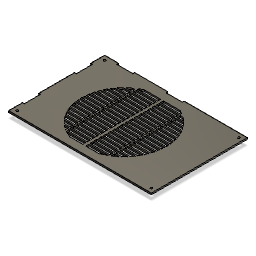
PSU and Board Enclosure (Autodesk Fusion 360 design; units mm, degrees)
Autodesk Fusion 360 part; units mm, degrees
note: some values were not read from the file. Chosen so that the rebuilt part matches the saved one: which bodies a step acts on; a direction; that a step has no effect; which face or edge a step refers to; which pieces of a blend or face edit are solid. Set by a fixed rule: which sketch regions a step uses.
(part 1 of 3)
mesh "Netz1" [no effect]
sketch "Skizze1" plane through (0, 0, 0) normal (0, 1, 0) x (1, 0, 0)
  line L0 (0, 0) -> (115, 0)
  line L1 (115, 0) -> (115, -240)
  line L2 (115, -240) -> (0, -240)
  line L3 (0, -240) -> (0, 0)
  line L4 (-7, 7) -> (122, 7)
  line L5 (122, 7) -> (122, -290)
  line L6 (122, -290) -> (-7, -290)
  line L7 (-7, -290) -> (-7, 7)
  line L8 (-9.4, 9.4) -> (124.4, 9.4)
  line L9 (124.4, 9.4) -> (124.4, -294)
  line L10 (124.4, -294) -> (-9.4, -294)
  line L11 (-9.4, -294) -> (-9.4, 9.4)
  line L12 (0, -240) -> (115, -240)
  line L13 (115, -240) -> (115, -290)
  line L14 (115, -290) -> (0, -290)
  line L15 (0, -290) -> (0, -240)
  line L16 (10, -225) -> (15, -225)
  line L17 (15, -225) -> (15, -230)
  line L18 (15, -230) -> (10, -230)
  line L19 (10, -230) -> (10, -225)
  line L20 (100, -225) -> (105, -225)
  line L21 (105, -225) -> (105, -230)
  line L22 (105, -230) -> (100, -230)
  line L23 (100, -230) -> (100, -225)
  line L24 (10, -120) -> (15, -120)
  line L25 (15, -120) -> (15, -125)
  line L26 (15, -125) -> (10, -125)
  line L27 (10, -125) -> (10, -120)
  line L28 (100, -120) -> (105, -120)
  line L29 (105, -120) -> (105, -125)
  line L30 (105, -125) -> (100, -125)
  line L31 (100, -125) -> (100, -120)
  line L32 (0, -25) -> (115, -25)
  line L33 (10, -40) -> (10, -35)
  line L34 (15, -40) -> (10, -40)
  line L35 (100, -40) -> (100, -35)
  line L36 (10, -35) -> (15, -35)
  line L37 (15, -35) -> (15, -40)
  line L38 (100, -35) -> (105, -35)
  line L39 (105, -40) -> (100, -40)
  line L40 (105, -35) -> (105, -40)
  circle A0 centre (40, -70) radius 30
  circle A1 centre (40, -70) radius 32.4
  line L41 (3.2857, -51.5) -> (78.5153, -51.5)
  line L42 (78.5153, -51.5) -> (78.5153, -56.5)
  line L43 (78.5153, -56.5) -> (3.2857, -56.5)
  line L44 (3.2857, -56.5) -> (3.2857, -51.5)
  line L45 (78.5153, -59.5) -> (78.5153, -64.5)
  line L46 (3.2857, -64.5) -> (3.2857, -59.5)
  line L47 (3.2857, -59.5) -> (78.5153, -59.5)
  line L48 (78.5153, -64.5) -> (3.2857, -64.5)
  line L49 (78.5153, -67.5) -> (78.5153, -72.5)
  line L50 (3.2857, -72.5) -> (3.2857, -67.5)
  line L51 (3.2857, -67.5) -> (78.5153, -67.5)
  line L52 (78.5153, -72.5) -> (3.2857, -72.5)
  line L53 (78.5153, -75.5) -> (78.5153, -80.5)
  line L54 (3.2857, -80.5) -> (3.2857, -75.5)
  line L55 (3.2857, -75.5) -> (78.5153, -75.5)
  line L56 (78.5153, -80.5) -> (3.2857, -80.5)
  line L57 (78.5153, -83.5) -> (78.5153, -88.5)
  line L58 (3.2857, -88.5) -> (3.2857, -83.5)
  line L59 (3.2857, -83.5) -> (78.5153, -83.5)
  line L60 (78.5153, -88.5) -> (3.2857, -88.5)
  line L61 (78.5153, -91.5) -> (78.5153, -96.5)
  line L62 (3.2857, -96.5) -> (3.2857, -91.5)
  line L63 (3.2857, -91.5) -> (78.5153, -91.5)
  line L64 (78.5153, -96.5) -> (3.2857, -96.5)
  line L65 (78.5153, -43.5) -> (78.5153, -48.5)
  line L66 (3.2857, -48.5) -> (3.2857, -43.5)
  line L67 (3.2857, -43.5) -> (78.5153, -43.5)
  line L68 (78.5153, -48.5) -> (3.2857, -48.5)
  dimension "d1" = 240
  dimension "d2" = 115
  dimension "d7" = 7
  dimension "d8" = 7
  dimension "d9" = 7
  dimension "d12" = 2.4
  dimension "d13" = 4
  dimension "d14" = 2.4
  dimension "d15" = 2.4
  dimension "d24" = 50
  dimension "d48" = 5
  dimension "d49" = 5
  dimension "d50" = 5
  dimension "d51" = 5
  dimension "d52" = 5
  dimension "d53" = 5
  dimension "d54" = 5
  dimension "d55" = 5
  dimension "d56" = 10
  dimension "d57" = 10
  dimension "d58" = 10
  dimension "d59" = 100
  dimension "d61" = 215
  dimension "d62" = 5
  dimension "d63" = 5
  dimension "d64" = 5
  dimension "d65" = 5
  dimension "d66" = 10
  dimension "d87" = 60
  dimension "d89" = 40
  dimension "d90" = 2.4
  dimension "d505" = 45
  dimension "d509" = 5
  dimension "d510" = 5
  dimension "d511" = 5
  dimension "d512" = 5
  dimension "d513" = 5
  dimension "d514" = 5
  dimension "d515" = 3
  dimension "d516" = 3
  dimension "d517" = 3
  dimension "d518" = 3
  dimension "d519" = 3
  dimension "d521" = 5
  dimension "d522" = 3
  dimension "d523" = 26.5
  constraint horizontal L0
  constraint vertical L1
  constraint horizontal L2
  constraint vertical L3
  constraint coincident L0.start L3.end
  constraint horizontal L4
  constraint vertical L5
  constraint horizontal L6
  constraint vertical L7
  constraint horizontal L8
  constraint vertical L9
  constraint horizontal L10
  constraint vertical L11
  constraint horizontal L12
  constraint vertical L13
  constraint horizontal L14
  constraint vertical L15
  constraint coincident L6 L14.end
  constraint horizontal L16
  constraint vertical L17
  constraint horizontal L18
  constraint vertical L19
  constraint horizontal L20
  constraint vertical L21
  constraint horizontal L22
  constraint vertical L23
  constraint horizontal L24
  constraint vertical L25
  constraint horizontal L26
  constraint vertical L27
  constraint horizontal L28
  constraint vertical L29
  constraint horizontal L30
  constraint vertical L31
  constraint horizontal L17.end L22.end
  constraint vertical L18.end L26.end
  constraint horizontal L26.end L30.end
  constraint vertical L22.end L30.end
  constraint coincident L3 L32.start
  constraint coincident L1 L32.end
  constraint perpendicular L1 L32
  constraint horizontal L36
  constraint vertical L37
  constraint horizontal L34
  constraint vertical L33
  constraint horizontal L38
  constraint vertical L40
  constraint horizontal L39
  constraint vertical L35
  constraint horizontal L35.start L33.start
  constraint vertical L26.end L33.start
  constraint vertical L30.end L35.start
  constraint concentric A0 A1
  constraint horizontal L41
  constraint vertical L42
  constraint horizontal L43
  constraint vertical L44
  constraint horizontal L47
  constraint vertical L45
  constraint horizontal L48
  constraint vertical L46
  constraint horizontal L51
  constraint vertical L49
  constraint horizontal L52
  constraint vertical L50
  constraint horizontal L55
  constraint vertical L53
  constraint horizontal L56
  constraint vertical L54
  constraint horizontal L59
  constraint vertical L57
  constraint horizontal L60
  constraint vertical L58
  constraint horizontal L63
  constraint vertical L61
  constraint horizontal L64
  constraint vertical L62
  constraint horizontal L67
  constraint vertical L65
  constraint horizontal L68
  constraint vertical L66
  measures "d1" distance of L0.start L2.end
  measures "d2" distance of L0.start L0.end
  measures "d7" distance of L3 L7
  measures "d8" distance of L1 L5
  measures "d9" distance of L0 L4
  measures "d12" distance of L5 L9
  measures "d13" distance of L6 L10
  measures "d14" distance of L7 L11
  measures "d15" distance of L4 L8
  measures "d24" distance of L2 L14.end
  measures "d48" distance of L16.start L16.end
  measures "d49" distance of L16.start L18.end
  measures "d50" distance of L20.start L20.end
  measures "d51" distance of L20.start L22.end
  measures "d52" distance of L24.start L24.end
  measures "d53" distance of L24.start L26.end
  measures "d54" distance of L28.start L28.end
  measures "d55" distance of L28.start L30.end
  measures "d56" distance of L3 L18.end
  measures "d57" distance of L1 L21.end
  measures "d58" distance of L12 L22
  measures "d59" vertical distance of L16.end L26.end
  measures "d61" distance of L2 L32
  measures "d62" distance of L36.end L33.end
  measures "d63" distance of L33.start L33.end
  measures "d64" distance of L35.end L38.end
  measures "d65" distance of L35.start L35.end
  measures "d66" distance of L32 L36.end
  measures "d87" diameter of A0
  measures "d89" distance of L3 A0.centre
  measures "d90" distance of A0 A1
  measures "d505" distance of L32 A0.centre
  measures "d509" distance of L41.start L43.end
  measures "d510" distance of L46.start L46.end
  measures "d511" distance of L50.start L50.end
  measures "d512" distance of L54.start L54.end
  measures "d513" distance of L58.start L58.end
  measures "d514" distance of L62.start L62.end
  measures "d515" distance of L60 L63
  measures "d516" distance of L56 L59
  measures "d517" distance of L52 L55
  measures "d518" distance of L48 L51
  measures "d519" distance of L43 L47
  measures "d521" distance of L66.start L66.end
  measures "d522" distance of L41 L66.start
  measures "d523" distance of A0.centre L67
sketch "Skizze24" plane through (0, 0, 0) normal (0, 1, 0) x (1, 0, 0)
  line L0 (8, -45) -> (107, -45)
  line L1 (107, -45) -> (107, -70)
  line L2 (107, -70) -> (8, -70)
  line L3 (8, -70) -> (8, -45)
  line L4 (8, -80) -> (107, -80)
  line L5 (107, -80) -> (107, -105)
  line L6 (107, -105) -> (8, -105)
  line L7 (8, -105) -> (8, -80)
  line L8 (8, -115) -> (107, -115)
  line L9 (107, -115) -> (107, -140)
  line L10 (107, -140) -> (8, -140)
  line L11 (8, -140) -> (8, -115)
  line L12 (8, -150) -> (107, -150)
  line L13 (107, -150) -> (107, -175)
  line L14 (107, -175) -> (8, -175)
  line L15 (8, -175) -> (8, -150)
  line L16 (8, -185) -> (107, -185)
  line L17 (107, -185) -> (107, -210)
  line L18 (107, -210) -> (8, -210)
  line L19 (8, -210) -> (8, -185)
  line L20 (8, -220) -> (107, -220)
  line L21 (107, -220) -> (107, -245)
  line L22 (107, -245) -> (8, -245)
  line L23 (8, -245) -> (8, -220)
  line L24 (0, 0) -> (115, 0)
  line L25 (115, -290) -> (0, -290)
  line L26 (-7, -290) -> (-7, 7)
  line L27 (122, 7) -> (122, -290)
  dimension "d486" = 45
  dimension "d487" = 45
  dimension "d488" = 25
  dimension "d489" = 25
  dimension "d490" = 25
  dimension "d491" = 25
  dimension "d492" = 25
  dimension "d493" = 25
  dimension "d494" = 10
  dimension "d495" = 10
  dimension "d496" = 10
  dimension "d497" = 10
  dimension "d498" = 20
  dimension "d503" = 15
  dimension "d504" = 15
  constraint horizontal L0
  constraint vertical L1
  constraint horizontal L2
  constraint vertical L3
  constraint horizontal L4
  constraint vertical L5
  constraint horizontal L6
  constraint vertical L7
  constraint horizontal L8
  constraint vertical L9
  constraint horizontal L10
  constraint vertical L11
  constraint horizontal L12
  constraint vertical L13
  constraint horizontal L14
  constraint vertical L15
  constraint horizontal L16
  constraint vertical L17
  constraint horizontal L18
  constraint vertical L19
  constraint horizontal L20
  constraint vertical L21
  constraint horizontal L22
  constraint vertical L23
  constraint vertical L2.end L6.end
  constraint vertical L6.end L10.end
  constraint vertical L12.start L16.start
  constraint vertical L10.end L12.start
  constraint vertical L18.end L20.start
  constraint vertical L17.end L20.end
  constraint vertical L13.end L16.end
  constraint vertical L9.end L12.end
  constraint vertical L5.end L8.end
  constraint vertical L1.end L4.end
  measures "d486" distance of L0 L24
  measures "d487" distance of L22 L25
  measures "d488" distance of L0 L2
  measures "d489" distance of L4 L6
  measures "d490" distance of L8 L10
  measures "d491" distance of L12 L14
  measures "d492" distance of L16 L18
  measures "d493" distance of L20 L22
  measures "d494" distance of L18 L20
  measures "d495" distance of L14 L16
  measures "d496" distance of L10 L12
  measures "d497" distance of L6 L8
  measures "d503" distance of L3 L26
  measures "d504" distance of L1 L27
extrude "Extrusion1" add sketch "Skizze1" along normal blind 2.4 contours L0 L1 L3 L4 L5 L6 L7 L13 L15 | L0 L1 L3 L32 | L1 L2 L3 L12 L32 | L2 L6 L12 L13 L14 L15 | L8 L9 L10 L11 | L16 L17 L18 L19 | L20 L21 L22 L23 | L24 L25 L26 L27 | L28 L29 L30 L31 | L33 L34 L36 L37 | L35 L38 L39 L40 | A0 L51 L52 | A0 A1 L51 L52 | A0 L48 L51 | A0 A1 L48 L51 | A0 A1 L52 L55 | A0 L52 L55 | A0 L47 L48 | A0 A1 L47 L48 | A0 A1 L48 L51 | A0 A1 L51 L52 | A1 L49 L51 L52 | A0 A1 L55 L56 | A0 L55 L56 | A0 A1 L52 L55 | A0 L43 L47 | A0 A1 L43 L47 | A1 L45 L47 L48 | A0 A1 L47 L48 | A1 L50 L51 L52 | A0 A1 L56 L59 | A0 L56 L59 | A0 A1 L55 L56 | A1 L53 L55 L56 | A0 L41 L43 | A0 A1 L41 L43 | A0 A1 L43 L47 | A1 L46 L47 L48 | A0 A1 L59 L60 | A0 L59 L60 | A0 A1 L56 L59 | A1 L54 L55 L56 | A0 L41 L68 | A0 A1 L41 L68 | A1 L41 L42 L43 | A0 A1 L41 L43 | A0 A1 L60 L63 | A0 L60 L63 | A0 A1 L59 L60 | A1 L57 L59 L60 | A0 L67 L68 | A0 A1 L67 L68 | A0 A1 L41 L68 | A1 L41 L43 L44 | A0 A1 L63 L64 | A0 L63 L64 | A0 A1 L60 L63 | A1 L58 L59 L60 | A0 L67 | A0 A1 L67 | A1 L65 L67 L68 | A0 A1 L67 L68 | A0 A1 L64 | A0 L64 | A0 A1 L63 L64 | A1 L61 L63 L64 | A1 L66 L67 L68 | A1 L62 L63 L64 makes body 1
extrude "Extrusion46" cut sketch "Skizze24" against normal up to surface (2.4 mm away) from surface at 2.4 bodies 1
extrude "Extrusion2" add sketch "Skizze1" along normal blind 64 from surface at 2.4 contours L8 L9 L10 L11 bodies 1
sketch "Skizze5" plane through (124.4, 0, 0) normal (1, 0, 0) x (0, 0, -1)
  line L0 (-294, 0) -> (9.4, 0)
  line L1 (9.4, 0) -> (9.4, 66.4)
  line L2 (9.4, 66.4) -> (-294, 66.4)
  line L3 (-294, 66.4) -> (-294, 0)
  line L4 (-40.6, 46) -> (-10.6, 46)
  line L5 (-10.6, 46) -> (-10.6, 41)
  line L6 (-10.6, 41) -> (-40.6, 41)
  line L7 (-40.6, 41) -> (-40.6, 46)
  line L8 (-40.6, 38) -> (-10.6, 38)
  line L9 (-10.6, 38) -> (-10.6, 33)
  line L10 (-10.6, 33) -> (-40.6, 33)
  line L11 (-40.6, 33) -> (-40.6, 38)
  line L12 (-40.6, 30) -> (-10.6, 30)
  line L13 (-10.6, 30) -> (-10.6, 25)
  line L14 (-10.6, 25) -> (-40.6, 25)
  line L15 (-40.6, 25) -> (-40.6, 30)
  line L16 (9.4, 0) -> (-294, 0)
  line L17 (-40.6, 22) -> (-10.6, 22)
  line L18 (-10.6, 22) -> (-10.6, 17)
  line L19 (-40.6, 17) -> (-40.6, 22)
  line L20 (-10.6, 17) -> (-40.6, 17)
  line L21 (-10.6, 14) -> (-10.6, 9)
  line L22 (-10.6, 9) -> (-40.6, 9)
  line L23 (-40.6, 9) -> (-40.6, 14)
  line L24 (-40.6, 14) -> (-10.6, 14)
  point P0 (-25, 0)
  dimension "d99" = 30
  dimension "d100" = 5
  dimension "d102" = 5
  dimension "d103" = 5
  dimension "d104" = 25
  dimension "d105" = 3
  dimension "d106" = 3
  dimension "d107" = 20
  dimension "d389" = 5
  dimension "d390" = 3
  dimension "d391" = 5
  dimension "d392" = 3
  constraint horizontal L4
  constraint vertical L5
  constraint horizontal L6
  constraint vertical L7
  constraint horizontal L8
  constraint vertical L9
  constraint horizontal L10
  constraint vertical L11
  constraint horizontal L12
  constraint vertical L13
  constraint horizontal L14
  constraint vertical L15
  constraint vertical L6.end L14.end
  constraint vertical L10.end L12.start
  constraint vertical L5.end L9.end
  constraint vertical L9.end L13.end
  constraint horizontal L17
  constraint vertical L18
  constraint horizontal L20
  constraint vertical L19
  constraint horizontal L24
  constraint vertical L21
  constraint horizontal L22
  constraint vertical L23
  constraint vertical L18.end L21.start
  constraint vertical L13.end L17.end
  constraint vertical L14.end L17.start
  constraint vertical L19.start L23.end
  measures "d99" distance of L4.start L4.end
  measures "d100" distance of L4.start L6.end
  measures "d102" distance of L8 L10
  measures "d103" distance of L12 L14
  measures "d104" distance of L14 L16
  measures "d105" distance of L10 L12
  measures "d106" distance of L6 L8
  measures "d107" distance of L1 L5.end
  measures "d389" distance of L17 L20
  measures "d390" distance of L14 L17
  measures "d391" distance of L22 L24
  measures "d392" distance of L20 L24
extrude "Extrusion12" cut sketch "Skizze5" against normal up to surface (133.8 mm away) contours L4 L5 L6 L7 | L8 L9 L10 L11 | L12 L13 L14 L15 | L17 L18 L19 L20 | L21 L22 L23 L24 bodies 1
extrude "Extrusion5" add sketch "Skizze1" along normal blind 50 from surface at 10 separate body contours L1 L2 L3 L12 L32 | L16 L17 L18 L19 | L20 L21 L22 L23 | L24 L25 L26 L27 | L28 L29 L30 L31 | L33 L34 L36 L37 | L35 L38 L39 L40 | A0 L51 L52 | A0 A1 L51 L52 | A0 L48 L51 | A0 A1 L48 L51 | A0 A1 L52 L55 | A0 L52 L55 | A0 L47 L48 | A0 A1 L47 L48 | A0 A1 L48 L51 | A0 A1 L51 L52 | A1 L49 L51 L52 | A0 A1 L55 L56 | A0 L55 L56 | A0 A1 L52 L55 | A0 L43 L47 | A0 A1 L43 L47 | A1 L45 L47 L48 | A0 A1 L47 L48 | A1 L50 L51 L52 | A0 A1 L56 L59 | A0 L56 L59 | A0 A1 L55 L56 | A1 L53 L55 L56 | A0 L41 L43 | A0 A1 L41 L43 | A0 A1 L43 L47 | A1 L46 L47 L48 | A0 A1 L59 L60 | A0 L59 L60 | A0 A1 L56 L59 | A1 L54 L55 L56 | A0 L41 L68 | A0 A1 L41 L68 | A1 L41 L42 L43 | A0 A1 L41 L43 | A0 A1 L60 L63 | A0 L60 L63 | A0 A1 L59 L60 | A1 L57 L59 L60 | A0 L67 L68 | A0 A1 L67 L68 | A0 A1 L41 L68 | A1 L41 L43 L44 | A0 A1 L63 L64 | A0 L63 L64 | A0 A1 L60 L63 | A1 L58 L59 L60 | A0 L67 | A0 A1 L67 | A1 L65 L67 L68 | A0 A1 L67 L68 | A0 A1 L64 | A0 L64 | A0 A1 L63 L64 | A1 L61 L63 L64 | A1 L66 L67 L68 | A1 L62 L63 L64 makes body 2
sketch "Skizze4" plane through (0, 0, 0) normal (-1, 0, 0) x (0, 0, 1)
  line L0 (25, 10) -> (240, 10)
  line L1 (240, 10) -> (240, 60)
  line L2 (240, 60) -> (25, 60)
  line L3 (25, 60) -> (25, 10)
  circle A0 centre (55, 25) radius 1.85
  circle A1 centre (205, 25) radius 1.85
  circle A2 centre (55, 25) radius 4.85
  circle A3 centre (205, 25) radius 4.85
  point P0 (25, 10)
  dimension "d69" = 3.7
  dimension "d70" = 3.7
  dimension "d71" = 150
  dimension "d72" = 30
  dimension "d73" = 35
  dimension "d76" = 3
  dimension "d77" = 3
  dimension "d502" = 15
  constraint horizontal A0.centre A1.centre
  constraint concentric A0 A2
  constraint concentric A1 A3
  measures "d69" diameter of A0
  measures "d70" diameter of A1
  measures "d71" distance of A0.centre A1.centre
  measures "d72" distance of L3 A0.centre
  measures "d73" distance of L1 A1.centre
  measures "d76" distance of A0 A2
  measures "d77" distance of A1 A3
  measures "d502" vertical distance of A0.centre P0
extrude "Extrusion8" cut sketch "Skizze4" against normal up to surface (133.8 mm away) from surface at 9.4 contours A0 | A1 bodies 1 2
extrude "Extrusion9" add sketch "Skizze4" against normal blind 6 from surface at 7 contours A2 | A3 bodies 1
extrude "Extrusion10" add sketch "Skizze4" along normal blind 6 from surface at -122 contours A2 | A3 bodies 1
chamfer "Fase1" distance 3 distance2 5.95 4 edges at (-7, 23.2462, 200.4782) (-7, 23.2462, 50.4782) (122, 26.7538, 200.4782) (122, 26.7538, 50.4782) measured on face at (-7, 31.5076, 263.2653) measured on face at (-7, 31.5076, 263.2653) measured on face at (122, 31.5076, 263.2653) measured on face at (122, 31.5076, 263.2653) on bodies 1
sketch "Skizze2" plane through (0, 0, 294) normal (0, 0, 1) x (1, 0, 0)
  line L0 (-9.4, 0) -> (124.4, 0)
  line L1 (124.4, 0) -> (124.4, 66.4)
  line L2 (124.4, 66.4) -> (-9.4, 66.4)
  line L3 (-9.4, 66.4) -> (-9.4, 0)
  line L4 (83.6, 39.9) -> (94.4, 39.9)
  line L5 (94.4, 39.9) -> (94.4, 10)
  line L6 (94.4, 10) -> (83.6, 10)
  line L7 (83.6, 10) -> (83.6, 39.9)
  line L8 (124.4, 0) -> (-9.4, 0)
  dimension "d25" = 10.8
  dimension "d26" = 29.9
  dimension "d39" = 30
  dimension "d40" = 10
  constraint horizontal L4
  constraint vertical L5
  constraint horizontal L6
  constraint vertical L7
  measures "d25" distance of L4.start L4.end
  measures "d26" distance of L4.start L6.end
  measures "d39" distance of L1 L5
  measures "d40" distance of L6 L8
sketch "Skizze3" plane through (0, 0, 294) normal (0, 0, 1) x (1, 0, 0)
  line L0 (-8.8, 65.8) -> (-8.8, 0)
  line L1 (33.7, 41) -> (6.2, 41)
  line L2 (6.2, 41) -> (6.2, 10)
  line L3 (6.2, 10) -> (33.7, 10)
  line L4 (33.7, 10) -> (33.7, 41)
  circle A0 centre (1.95, 25.5) radius 1.25
  circle A1 centre (37.95, 25.5) radius 1.25
  line L5 (-9.4, 0) -> (124.4, 0)
  line L6 (124.4, 0) -> (124.4, 66.4)
  line L7 (124.4, 66.4) -> (-9.4, 66.4)
  line L8 (-9.4, 66.4) -> (-9.4, 0)
  line L9 (124.4, 0) -> (-9.4, 0)
  line L10 (33.7, 35.5) -> (28.2, 41)
  line L11 (11.7, 41) -> (6.2, 35.5)
  dimension "d27" = 27.5
  dimension "d28" = 31
  dimension "d29" = 2.5
  dimension "d30" = 2.5
  dimension "d32" = 36
  dimension "d33" = 15.5
  dimension "d44" = 15
  dimension "d45" = 10
  dimension "d393" = 4.25
  dimension "d394" = 2.9455
  dimension "d396" = 25.5
  dimension "d397" = 16.5
  dimension "d398" = 5.5
  constraint horizontal L1
  constraint vertical L2
  constraint horizontal L3
  constraint vertical L4
  constraint horizontal A0.centre A1.centre
  constraint coincident L4 L10.start
  constraint coincident L1 L10.end
  constraint coincident L1 L11.start
  constraint coincident L2 L11.end
  constraint horizontal L10.start L11.end
  measures "d27" distance of L1.start L1.end
  measures "d28" distance of L1.start L3.end
  measures "d29" diameter of A0
  measures "d30" diameter of A1
  measures "d32" distance of A0.centre A1.centre
  measures "d33" distance of L1 A0.centre
  measures "d44" distance of L0 L2
  measures "d45" distance of L3 L9
  measures "d393" distance of L2 A0.centre
  measures "d396" distance of L3 L11.end
  measures "d397" distance of L10.end L11.start
  measures "d398" distance of L1.end L11.start
extrude "Extrusion4" cut sketch "Skizze2" against normal up to surface (4 mm away) contours L4 L5 L6 L7 bodies 1
extrude "Extrusion6" cut sketch "Skizze3" against normal up to surface (4 mm away) contours L1 L2 L3 L4 L10 L11 | A0 | A1 bodies 1
fillet "Abrundung3" radius 1.5 2 edges at (6.2, 10, 292) (33.7, 10, 292) on bodies 1
sketch "Skizze6" plane through (-7, 0, 0) normal (1, 0, 0) x (0, 0, -1)
  line L0 (-41.2, 51) -> (-41.2, 56)
  line L1 (-41.2, 56) -> (-11.2, 56)
  line L2 (-11.2, 56) -> (-11.2, 51)
  line L3 (-11.2, 51) -> (-41.2, 51)
  line L4 (-41.2, 43) -> (-41.2, 48)
  line L5 (-41.2, 48) -> (-11.2, 48)
  line L6 (-11.2, 48) -> (-11.2, 43)
  line L7 (-11.2, 43) -> (-41.2, 43)
  line L8 (-41.2, 35) -> (-41.2, 40)
  line L9 (-41.2, 40) -> (-11.2, 40)
  line L10 (-11.2, 40) -> (-11.2, 35)
  line L11 (-11.2, 35) -> (-41.2, 35)
  circle A0 centre (-55, 42) radius 1.85
  circle A1 centre (-205, 42) radius 1.85
  line L12 (-294, 0) -> (8.8, 0)
  line L13 (8.8, 0) -> (8.8, 65.8)
  line L14 (8.8, 65.8) -> (-294, 65.8)
  line L15 (-294, 65.8) -> (-294, 0)
  line L16 (-269, 65.8) -> (-249, 65.8)
  line L17 (-249, 65.8) -> (-249, 75.8)
  line L18 (-249, 75.8) -> (-269, 75.8)
  line L19 (-269, 75.8) -> (-269, 65.8)
  line L20 (-151.2, 65.8) -> (-131.2, 65.8)
  line L21 (-131.2, 65.8) -> (-131.2, 75.8)
  line L22 (-131.2, 75.8) -> (-151.2, 75.8)
  line L23 (-151.2, 75.8) -> (-151.2, 65.8)
  line L24 (-16.2, 65.8) -> (-36.2, 65.8)
  line L25 (-36.2, 65.8) -> (-36.2, 75.8)
  line L26 (-36.2, 75.8) -> (-16.2, 75.8)
  line L27 (-16.2, 75.8) -> (-16.2, 65.8)
  circle A2 centre (-259, 70.8) radius 2.05
  circle A3 centre (-141.2, 70.8) radius 2.05
  circle A4 centre (-26.2, 70.8) radius 2.05
  line L28 (-40.6, 41) -> (-40.6, 46)
  line L29 (-40.6, 46) -> (-10.6, 46)
  line L30 (-10.6, 46) -> (-10.6, 41)
  line L31 (-10.6, 41) -> (-40.6, 41)
  line L32 (-40.6, 33) -> (-40.6, 38)
  line L33 (-40.6, 38) -> (-10.6, 38)
  line L34 (-10.6, 38) -> (-10.6, 33)
  line L35 (-10.6, 33) -> (-40.6, 33)
  line L36 (-40.6, 25) -> (-40.6, 30)
  line L37 (-40.6, 30) -> (-10.6, 30)
  line L38 (-10.6, 30) -> (-10.6, 25)
  line L39 (-10.6, 25) -> (-40.6, 25)
  line L40 (-290, 2.4) -> (7, 2.4)
  line L41 (7, 2.4) -> (7, 66.4)
  line L42 (7, 66.4) -> (-290, 66.4)
  line L43 (-290, 66.4) -> (-290, 2.4)
  line L44 (-10.6, 17) -> (-40.6, 17)
  line L45 (-40.6, 17) -> (-40.6, 22)
  line L46 (-40.6, 22) -> (-10.6, 22)
  line L47 (-10.6, 22) -> (-10.6, 17)
  line L48 (-40.6, 14) -> (-10.6, 14)
  line L49 (-10.6, 14) -> (-10.6, 9)
  line L50 (-10.6, 9) -> (-40.6, 9)
  line L51 (-40.6, 9) -> (-40.6, 14)
  circle A5 centre (-205, 25) radius 7.85
  circle A6 centre (-55, 25) radius 7.85
  point P0 (-294, 65.8)
  dimension "d111" = 20
  dimension "d112" = 10
  dimension "d113" = 20
  dimension "d114" = 10
  dimension "d115" = 20
  dimension "d116" = 10
  dimension "d117" = 25
  dimension "d118" = 25
  dimension "d120" = 140
  dimension "d128" = 4.1
  dimension "d129" = 10
  dimension "d130" = 5
  dimension "d131" = 4.1
  dimension "d132" = 10
  dimension "d133" = 5
  dimension "d134" = 4.1
  dimension "d135" = 10
  dimension "d136" = 5
  dimension "d285" = 10
  dimension "d287" = 10
  constraint horizontal L16
  constraint vertical L17
  constraint horizontal L18
  constraint vertical L19
  constraint coincident L14 L16.start
  constraint horizontal L20
  constraint vertical L21
  constraint horizontal L22
  constraint vertical L23
  constraint coincident L14 L20.start
  constraint horizontal L24
  constraint vertical L25
  constraint horizontal L26
  constraint vertical L27
  constraint coincident L14 L24.start
  measures "d111" distance of L16.start L16.end
  measures "d112" distance of L16.start L18.end
  measures "d113" distance of L20.start L20.end
  measures "d114" distance of L20.start L22.end
  measures "d115" distance of L24.start L24.end
  measures "d116" distance of L24.start L26.end
  measures "d117" distance of L19 P0
  measures "d118" distance of L13.end L27
  measures "d120" distance of L13.end L21
  measures "d128" diameter of A2
  measures "d129" distance of L19 A2.centre
  measures "d130" distance of L16 A2.centre
  measures "d131" diameter of A3
  measures "d132" distance of L23 A3.centre
  measures "d133" distance of L20 A3.centre
  measures "d134" diameter of A4
  measures "d135" distance of L25 A4.centre
  measures "d136" distance of L24 A4.centre
extrude "Extrusion13" add sketch "Skizze6" against normal up to surface (2.4 mm away) contours L17 L18 L19 L42 | L25 L26 L27 L42 | L21 L22 L23 L42 bodies 1
sketch "Skizze7" plane through (0, 0, 294) normal (0, 0, 1) x (1, 0, 0)
  line L0 (0.6, 65.8) -> (20.6, 65.8)
  line L1 (20.6, 65.8) -> (20.6, 75.8)
  line L2 (20.6, 75.8) -> (0.6, 75.8)
  line L3 (0.6, 75.8) -> (0.6, 65.8)
  circle A0 centre (10.6, 70.8) radius 2.05
  line L4 (94.4, 75.8) -> (114.4, 75.8)
  line L5 (114.4, 75.8) -> (114.4, 65.8)
  line L6 (114.4, 65.8) -> (94.4, 65.8)
  line L7 (94.4, 65.8) -> (94.4, 75.8)
  line L8 (124.4, 0) -> (124.4, 66.4)
  circle A1 centre (104.4, 70.8) radius 2.05
  point P0 (-8.8, 65.8)
  point P1 (-9.4, 66.4)
  point P2 (-7, 65.8)
  dimension "d137" = 20
  dimension "d138" = 10
  dimension "d139" = 4.1
  dimension "d140" = 10
  dimension "d141" = 5
  dimension "d142" = 10
  dimension "d143" = 20
  dimension "d144" = 10
  dimension "d145" = 10
  dimension "d146" = 4.1
  dimension "d147" = 10
  dimension "d148" = 5
  constraint horizontal L0
  constraint vertical L1
  constraint horizontal L2
  constraint vertical L3
  constraint coincident L0 P0
  constraint horizontal L4
  constraint vertical L5
  constraint horizontal L6
  constraint vertical L7
  constraint coincident L6 P2
  measures "d137" distance of L1.end L2.end
  measures "d138" distance of L0.start L2.end
  measures "d139" diameter of A0
  measures "d140" distance of L3 A0.centre
  measures "d141" distance of L0 A0.centre
  measures "d142" horizontal distance of L2.end P1
  measures "d143" distance of L4.start L4.end
  measures "d144" distance of L4.start L6.end
  measures "d145" distance of L5 L8
  measures "d146" diameter of A1
  measures "d147" distance of L7 A1.centre
  measures "d148" distance of L6 A1.centre
extrude "Extrusion15" add sketch "Skizze7" against normal up to surface (4 mm away) bodies 1
sketch "Skizze8" plane through (0, 66.4, 0) normal (0, 1, 0) x (-1, 0, 0)
  line L0 (9.4, 131.2) -> (7, 131.2)
  line L1 (7, 131.2) -> (7, 36.2)
  line L2 (7, 36.2) -> (9.4, 36.2)
  line L3 (9.4, 36.2) -> (9.4, 131.2)
  line L4 (9.4, -9.4) -> (-124.4, -9.4)
  line L5 (-124.4, -9.4) -> (-124.4, 294)
  line L6 (-124.4, 294) -> (9.4, 294)
  line L7 (9.4, 294) -> (9.4, -9.4)
  line L8 (-124.4, 294) -> (9.4, 294)
  line L9 (-124.4, 249) -> (9.4, 249)
  line L10 (9.4, 249) -> (9.4, 269)
  line L11 (9.4, 269) -> (-124.4, 269)
  line L12 (-124.4, 269) -> (-124.4, 249)
  line L13 (7, 249) -> (9.4, 249)
  line L14 (7, 269) -> (9.4, 269)
  line L15 (-114.4, 294) -> (-94.4, 294)
  line L16 (-94.4, 294) -> (-94.4, 290)
  line L17 (-94.4, 290) -> (-114.4, 290)
  line L18 (-114.4, 290) -> (-114.4, 294)
  line L19 (-0.6, 290) -> (-20.6, 290)
  line L20 (-20.6, 290) -> (-20.6, 294)
  line L21 (-20.6, 294) -> (-0.6, 294)
  line L22 (-0.6, 294) -> (-0.6, 290)
  line L23 (-0.6, 294) -> (-0.6, 290)
  line L24 (-20.6, 294) -> (-20.6, 290)
  line L25 (-94.4, 290) -> (-114.4, 290)
  line L26 (-114.4, 294) -> (-114.4, 290)
  line L27 (9.4, 131.2) -> (7, 131.2)
  line L28 (7, 131.2) -> (7, 151.2)
  line L29 (7, 151.2) -> (9.4, 151.2)
  line L30 (9.4, 151.2) -> (9.4, 131.2)
  line L31 (9.4, 16.2) -> (-124.4, 16.2)
  line L32 (-124.4, 16.2) -> (-124.4, 36.2)
  line L33 (-124.4, 36.2) -> (9.4, 36.2)
  line L34 (9.4, 36.2) -> (9.4, 16.2)
  line L35 (4.6, 287.6) -> (-119.6, 287.6)
  line L36 (-119.6, 287.6) -> (-119.6, -4.6)
  line L37 (-119.6, -4.6) -> (4.6, -4.6)
  line L38 (4.6, -4.6) -> (4.6, 287.6)
  line L39 (7, -7) -> (-122, -7)
  line L40 (-122, -7) -> (-122, 290)
  line L41 (7, 290) -> (7, -7)
  line L42 (-115, 290) -> (0, 290)
  line L43 (7, 290) -> (-122, 290)
  line L44 (-122, 290) -> (-122, -7)
  line L45 (-122, -7) -> (7, -7)
  line L46 (7, -7) -> (7, 290)
  point P0 (-124.4, -9.4)
  point P1 (9.4, -9.4)
  point P2 (-94.4, 294)
  point P3 (7, 151.2)
  point P4 (9.4, 16.2)
  dimension "d158" = 2.4
  dimension "d159" = 2.4
  dimension "d160" = 2.4
  dimension "d161" = 2.4
  constraint horizontal L4
  constraint vertical L5
  constraint horizontal L6
  constraint vertical L7
  constraint coincident P0 L4.end
  constraint coincident P1 L4.start
  constraint coincident L6.end L8
  constraint horizontal L9
  constraint vertical L10
  constraint horizontal L11
  constraint vertical L12
  constraint coincident L5 L9.start
  constraint coincident L9.start L13
  constraint coincident L9.end L10.start
  constraint coincident L11.end L14
  constraint horizontal L15
  constraint vertical L16
  constraint horizontal L17
  constraint vertical L18
  constraint horizontal L19
  constraint vertical L20
  constraint horizontal L21
  constraint vertical L22
  constraint coincident L19.start L23
  constraint coincident L19.end L24
  constraint coincident L19 L20.start
  constraint coincident L21 L20.end
  constraint coincident L16.end L25
  constraint coincident P2 L15.end
  constraint coincident L15.start L26
  constraint horizontal L27
  constraint vertical L28
  constraint horizontal L29
  constraint vertical L30
  constraint coincident L0.start L3.end
  constraint coincident L29 P3
  constraint coincident L28 P3
  constraint horizontal L31
  constraint vertical L32
  constraint horizontal L33
  constraint vertical L34
  constraint coincident P4 L31.start
  constraint coincident L5 L31.end
  constraint coincident L1.end L33
  constraint horizontal L35
  constraint vertical L36
  constraint horizontal L37
  constraint vertical L38
  constraint horizontal L43
  constraint vertical L44
  constraint horizontal L45
  constraint vertical L46
  constraint coincident L39.end L40.start
  constraint coincident L41.start L43.start
  measures "d158" distance of L37 L39
  measures "d159" distance of L36 L40
  measures "d160" distance of L38 L41
  measures "d161" distance of L35 L42
extrude "Extrusion17" add sketch "Skizze8" along normal blind 2 from surface at 5 separate body contours L0 L1 L2 L3 L7 L27 L33 L41 L46 | L1 L9 L28 L33 L38 L41 L46 | L7 L9 L13 L29 L41 L46 | L31 L33 L38 L41 L46 | L4 L5 L7 L31 L39 L40 L41 L44 L45 L46 | L31 L33 L36 L38 | L9 L33 L36 L38 | L31 L36 L37 L38 L39 L40 L41 L44 L45 L46 | L9 L11 L38 L41 L46 | L6 L7 L8 L11 L14 L22 L23 L41 L42 L43 L46 | L31 L33 L36 L40 L44 | L9 L33 L36 L40 L44 | L31 L36 L37 L38 | L9 L11 L36 L38 | L11 L17 L19 L25 L35 L36 L38 L40 L41 L42 L43 L44 L46 | L5 L31 L32 L33 L40 L44 | L5 L9 L33 L40 L44 | L9 L11 L36 L40 L44 | L11 L35 L36 L38 | L5 L9 L11 L12 L40 L44 | L6 L8 L16 L20 L24 L42 L43 | L5 L6 L8 L11 L18 L26 L40 L42 L43 L44 makes body 3
extrude "Extrusion18" add sketch "Skizze8" against normal blind 1 from surface at 5 contours L1 L9 L28 L33 L38 L41 L46 | L31 L33 L38 L41 L46 | L31 L36 L37 L38 L39 L40 L41 L44 L45 L46 | L9 L11 L38 L41 L46 | L31 L33 L36 L40 L44 | L9 L33 L36 L40 L44 | L11 L17 L19 L25 L35 L36 L38 L40 L41 L42 L43 L44 L46 | L9 L11 L36 L40 L44 bodies 3
extrude "Extrusion48" cut sketch "Skizze1" against normal up to surface (2 mm away) from surface at 73.4 contours A0 L51 L52 | A0 L47 L48 | A0 L55 L56 | A0 L41 L43 | A0 L59 L60 | A0 L67 L68 | A0 L63 L64 bodies 3
fillet "Abrundung1" radius 1 12 edges at (-7, 70.4, 141.5) (57.5, 70.4, 290) (-8.2, 71.4, 249) (20.6, 71.4, 292) (94.4, 71.4, 292) (0.6, 71.4, 292) (-8.2, 71.4, 151.2) (-8.2, 71.4, 269) (-8.2, 71.4, 36.2) (-8.2, 71.4, 131.2) (-8.2, 71.4, 16.2) (114.4, 71.4, 292) on bodies 3
sketch "Skizze22" plane through (0, 66.4, 0) normal (0, 1, 0) x (-1, 0, 0)
  line L0 (-114.4, 290) -> (-114.4, 294)
  line L1 (-114.4, 294) -> (-124.4, 294)
  line L2 (-124.4, 294) -> (-124.4, -9.4)
  line L3 (-124.4, -9.4) -> (9.4, -9.4)
  line L4 (9.4, -9.4) -> (9.4, 16.2)
  line L5 (9.4, 16.2) -> (7, 16.2)
  line L6 (7, 16.2) -> (7, -7)
  line L7 (7, -7) -> (-122, -7)
  line L8 (-122, -7) -> (-122, 290)
  line L9 (-122, 290) -> (-114.4, 290)
  line L10 (4.6, -4.6) -> (-119.6, -4.6)
  line L11 (-119.6, -4.6) -> (-119.6, 287.6)
  line L12 (-119.6, 287.6) -> (4.6, 287.6)
  line L13 (4.6, 287.6) -> (4.6, -4.6)
  line L14 (-122, -7) -> (-122, 290)
  line L15 (-122, 290) -> (7, 290)
  line L16 (7, 290) -> (7, -7)
  line L17 (7, -7) -> (-122, -7)
  dimension "d444" = 2.4
  dimension "d445" = 2.4
  dimension "d446" = 2.4
  dimension "d447" = 4
  dimension "d448" = 2.4
  constraint horizontal L10
  constraint vertical L11
  constraint horizontal L12
  constraint vertical L13
  measures "d444" distance of L11 L14
  measures "d445" distance of L12 L15
  measures "d446" distance of L13 L16
  measures "d448" distance of L10 L17
extrude "Extrusion37" add sketch "Skizze22" against normal blind 2.4 from surface at -10 contours L6 L7 L8 L9 L14 L15 L16 L17 bodies 1
sketch "Skizze9" plane through (0, 0, 0) normal (0, 1, 0) x (1, 0, 0)
  line L0 (-9.4, 160.2) -> (185, 160.2)
  line L1 (185, 160.2) -> (185, 29.4)
  line L2 (185, 29.4) -> (-9.4, 29.4)
  line L3 (-9.4, 29.4) -> (-9.4, 160.2)
  line L4 (160, 61.8) -> (13, 61.8)
  line L5 (13, 61.8) -> (13, 156.8)
  line L6 (13, 156.8) -> (160, 156.8)
  line L7 (160, 156.8) -> (160, 61.8)
  circle A0 centre (155.5, 66.3) radius 1.5
  circle A1 centre (155.5, 152.3) radius 1.5
  circle A2 centre (17.5, 66.3) radius 1.5
  circle A3 centre (17.5, 152.3) radius 1.5
  line L8 (84.55, 156.8) -> (68.35, 156.8)
  line L9 (68.35, 156.8) -> (68.35, 151.8)
  line L10 (68.35, 151.8) -> (84.55, 151.8)
  line L11 (84.55, 151.8) -> (84.55, 156.8)
  line L12 (68.35, 156.8) -> (49.9, 156.8)
  line L13 (49.9, 156.8) -> (49.9, 151.8)
  line L14 (49.9, 151.8) -> (68.35, 151.8)
  line L15 (68.35, 151.8) -> (68.35, 156.8)
  line L16 (182.6, 31.8) -> (-7, 31.8)
  line L17 (-7, 31.8) -> (-7, 157.8)
  line L18 (-7, 157.8) -> (182.6, 157.8)
  line L19 (182.6, 157.8) -> (182.6, 31.8)
  circle A4 centre (17.5, 152.3) radius 3.5
  circle A5 centre (155.5, 152.3) radius 3.5
  circle A6 centre (155.5, 66.3) radius 3.5
  circle A7 centre (17.5, 66.3) radius 3.5
  line L20 (49.9, 156.8) -> (31.68, 156.8)
  line L21 (31.68, 156.8) -> (31.68, 151.8)
  line L22 (31.68, 151.8) -> (49.9, 151.8)
  line L23 (49.9, 151.8) -> (49.9, 156.8)
  line L24 (48.9, 156.8) -> (48.9, 151.8)
  line L25 (48.9, 151.8) -> (50.9, 151.8)
  line L26 (50.9, 151.8) -> (50.9, 156.8)
  line L27 (50.9, 156.8) -> (48.9, 156.8)
  line L28 (67.35, 156.8) -> (67.35, 151.8)
  line L29 (69.35, 151.8) -> (69.35, 156.8)
  line L30 (69.35, 156.8) -> (67.35, 156.8)
  circle A8 centre (-3.5, 35.3) radius 1.5
  circle A9 centre (-3.5, 35.3) radius 3.5
  circle A10 centre (-3.5, 154.3) radius 1.5
  circle A11 centre (-3.5, 154.3) radius 3.5
  circle A12 centre (179.1, 154.3) radius 1.5
  circle A13 centre (179.1, 154.3) radius 3.5
  circle A14 centre (179.1, 35.3) radius 3.5
  circle A15 centre (179.1, 35.3) radius 1.5
  line L31 (-7, 31.8) -> (-7, 38.8)
  line L32 (-7, 38.8) -> (0, 38.8)
  line L33 (0, 38.8) -> (0, 31.8)
  line L34 (0, 31.8) -> (-7, 31.8)
  line L35 (-7, 157.8) -> (-7, 150.8)
  line L36 (-7, 150.8) -> (0, 150.8)
  line L37 (0, 150.8) -> (0, 157.8)
  line L38 (0, 157.8) -> (-7, 157.8)
  line L39 (182.6, 157.8) -> (182.6, 150.8)
  line L40 (182.6, 150.8) -> (175.6, 150.8)
  line L41 (175.6, 150.8) -> (175.6, 157.8)
  line L42 (175.6, 157.8) -> (182.6, 157.8)
  line L43 (175.6, 31.8) -> (175.6, 38.8)
  line L44 (175.6, 38.8) -> (182.6, 38.8)
  line L45 (182.6, 38.8) -> (182.6, 31.8)
  line L46 (182.6, 31.8) -> (175.6, 31.8)
  line L47 (-9.4, 9.4) -> (124.4, 9.4)
  line L48 (-2, 116.8) -> (8, 116.8)
  line L49 (8, 116.8) -> (8, 96.8)
  line L50 (8, 96.8) -> (-2, 96.8)
  line L51 (-2, 96.8) -> (-2, 116.8)
  point P0 (-9.4, 9.4)
  dimension "d169" = 147
  dimension "d170" = 95
  dimension "d171" = 3
  dimension "d173" = 3
  dimension "d174" = 3
  dimension "d175" = 3
  dimension "d177" = 4.5
  dimension "d179" = 4.5
  dimension "d180" = 16.2
  dimension "d181" = 5
  dimension "d182" = 75.45
  dimension "d183" = 18.45
  dimension "d184" = 5
  dimension "d190" = 2.4
  dimension "d191" = 2.4
  dimension "d192" = 2.4
  dimension "d193" = 2.4
  dimension "d197" = 2
  dimension "d198" = 2
  dimension "d199" = 2
  dimension "d200" = 2
  dimension "d204" = 20
  dimension "d228" = 208.8
  dimension "d232" = 18.22
  dimension "d240" = 1
  dimension "d241" = 30
  dimension "d242" = 4.5
  dimension "d243" = 4.5
  dimension "d245" = 2
  dimension "d246" = 1
  dimension "d247" = 2
  dimension "d248" = 1
  dimension "d635" = 3
  dimension "d637" = 2
  dimension "d638" = 3
  dimension "d639" = 2
  dimension "d640" = 3
  dimension "d641" = 2
  dimension "d642" = 3
  dimension "d643" = 2
  dimension "d662" = 20
  dimension "d663" = 194.4
  dimension "d664" = 10
  dimension "d665" = 20
  dimension "d666" = 5
  dimension "d667" = 40
  constraint coincident L6 L8.start
  constraint concentric A3 A4
  constraint concentric A1 A5
  constraint concentric A0 A6
  constraint concentric A2 A7
  constraint coincident L13.end L22
  constraint perpendicular L0 L1
  constraint perpendicular L1 L16
  constraint perpendicular L2 L3
  constraint perpendicular L12 L13
  constraint perpendicular L10 L11
  constraint perpendicular L14 L15
  constraint perpendicular L8 L9
  constraint perpendicular L6 L11
  constraint perpendicular L21 L22
  constraint perpendicular L22 L23
  constraint perpendicular L8 L11
  constraint parallel L6 L14
  constraint parallel L6 L20
  constraint perpendicular L20 L21
  constraint coincident L14 L25.end
  constraint coincident L20 L24.start
  constraint coincident L10 L29.start
  constraint coincident L12 L28.start
  constraint concentric A8 A9
  constraint tangent L16 A9
  constraint tangent L17 A9
  constraint concentric A10 A11
  constraint tangent L17 A11
  constraint tangent L18 A11
  constraint concentric A12 A13
  constraint tangent L19 A13
  constraint tangent L18 A13
  constraint concentric A14 A15
  constraint tangent L16 A14
  constraint tangent L19 A14
  constraint tangent A9 L32
  constraint tangent A9 L33
  constraint tangent A11 L37
  constraint tangent A11 L36
  constraint tangent A13 L41
  constraint tangent A13 L40
  constraint coincident L19 L44.end
  constraint coincident L16 L43.start
  constraint tangent A14 L43
  constraint tangent A14 L44
  constraint coincident L3 P0
  constraint perpendicular L32 L33
  constraint perpendicular L31 L32
  constraint perpendicular L16 L33
  constraint perpendicular L43 L44
  constraint perpendicular L16 L43
  constraint perpendicular L41 L42
  constraint perpendicular L40 L41
  constraint perpendicular L39 L40
  constraint perpendicular L18 L41
  constraint perpendicular L36 L37
  constraint perpendicular L17 L36
  constraint horizontal A1.centre A3.centre
  constraint vertical A1.centre A0.centre
  constraint horizontal A0.centre A2.centre
  constraint vertical A3.centre A2.centre
  constraint perpendicular L4 L7
  constraint horizontal L48
  constraint vertical L49
  constraint horizontal L50
  constraint vertical L51
  measures "d169" distance of L4.start L4.end
  measures "d170" distance of L4.start L6.end
  measures "d171" diameter of A0
  measures "d173" diameter of A1
  measures "d174" diameter of A2
  measures "d175" diameter of A3
  measures "d177" distance of L5 A2.centre
  measures "d179" distance of L6 A3.centre
  measures "d180" distance of L8.start L8.end
  measures "d181" distance of L8.start L10.end
  measures "d182" distance of L6.end L11
  measures "d183" distance of L8.end L12.end
  measures "d184" distance of L12 L14
  measures "d190" distance of L0 L18
  measures "d191" distance of L1 L19
  measures "d192" distance of L3 L17
  measures "d193" distance of L2 L16
  measures "d197" distance of A3 A4
  measures "d198" distance of A1 A5
  measures "d199" distance of A0 A6
  measures "d200" distance of A2 A7
  measures "d204" distance of L5 L17
  measures "d232" distance of L12.end L20.end
  measures "d240" distance of L6 L18
  measures "d241" distance of L4 L16
  measures "d242" distance of L7 A0.centre
  measures "d243" distance of L4 A2.centre
  measures "d245" distance of L24 L26
  measures "d246" distance of L13 L26
  measures "d247" distance of L28 L29
  measures "d248" distance of L9 L28
  measures "d635" diameter of A8
  measures "d637" distance of A8 A9
  measures "d638" diameter of A10
  measures "d639" distance of A10 A11
  measures "d640" diameter of A12
  measures "d641" distance of A12 A13
  measures "d642" diameter of A15
  measures "d643" distance of A14 A15
  measures "d662" distance of L2 L47
  measures "d663" distance of L1 L3
  measures "d664" distance of L48.start L48.end
  measures "d665" distance of L48.start L50.end
  measures "d666" distance of L17 L51
  measures "d667" distance of L6 L48
extrude "SKR-Gehäuse" add sketch "Skizze9" against normal blind 2.4 separate body contours L0 L1 L2 L3 | L4 L5 L6 L7 L10 L11 L14 L21 L22 L25 | L6 L8 L10 L11 L29 | L6 L20 L21 L22 L24 | L6 L8 L9 L10 L15 L29 L30 | L6 L13 L20 L22 L23 L24 L25 L27 | L6 L9 L12 L14 L15 L28 L30 | L6 L12 L13 L14 L23 L25 L26 L27 | L6 L12 L14 L26 L28 | L16 A14 L43 L46 | L16 L17 L18 L19 L32 L33 L36 L37 L40 L41 L43 L44 | L16 A9 L33 L34 | L16 L19 A14 L45 L46 | A14 | A14 L43 L44 | L16 L17 A9 L31 L34 | A9 | A9 L32 L33 | L19 A14 L44 L45 | L17 A9 L31 L32 | L19 A13 L39 L40 | L17 A11 L35 L36 | L18 L19 A13 L39 L42 | A13 | A13 L40 L41 | L17 L18 A11 L35 L38 | A11 | A11 L36 L37 | L18 A13 L41 L42 | L18 A11 L37 L38 | A4 | A5 | A6 | A7 makes body 4
extrude "Extrusion20" add sketch "Skizze9" along normal blind 90 separate body contours L0 L1 L2 L3 makes body 5
extrude "Extrusion61" add sketch "Skizze9" along normal blind 10 contours L16 A14 L43 L46 | L16 A9 L33 L34 | L16 L19 A14 L45 L46 | A14 | L16 L17 A9 L31 L34 | A9 | L19 A14 L44 L45 | L17 A9 L31 L32 | L19 A13 L39 L40 | L17 A11 L35 L36 | L18 L19 A13 L39 L42 | A13 | L17 L18 A11 L35 L38 | A11 | L18 A13 L41 L42 | L18 A11 L37 L38 bodies 5
extrude "Extrusion21" add sketch "Skizze9" along normal blind 10 contours A4 | A5 | A6 | A7 bodies 4
extrude "Extrusion57" add sketch "Skizze9" against normal blind 20 from surface at 87.5 contours L16 A14 L43 L46 | L16 A9 L33 L34 | L16 L19 A14 L45 L46 | A14 | A14 L43 L44 | L16 L17 A9 L31 L34 | A9 | A9 L32 L33 | L19 A14 L44 L45 | L17 A9 L31 L32 | L19 A13 L39 L40 | L17 A11 L35 L36 | L18 L19 A13 L39 L42 | A13 | A13 L40 L41 | L17 L18 A11 L35 L38 | A11 | A11 L36 L37 | L18 A13 L41 L42 | L18 A11 L37 L38 | A8 | A10 | A12 | A15 bodies 2 3 1 5 4
chamfer "Fase9" distance 6.7 distance2 4.5 4 edges at (-3.5, 67.5, -38.8) (-3.5, 67.5, -150.8) (179.1, 67.5, -38.8) (179.1, 67.5, -150.8) measured on face at (-4.6667, 67.5, -34.1333) measured on face at (-4.6667, 67.5, -155.4667) measured on face at (180.2667, 67.5, -34.1333) measured on face at (177.9333, 67.5, -155.4667) on bodies 5
fillet "Abrundung4" radius 3.5 4 edges at (0, 79.75, -38.8) (175.6, 79.75, -38.8) (175.6, 79.75, -150.8) (0, 79.75, -150.8) on bodies 5
extrude "Extrusion58" cut sketch "Skizze9" against normal blind 15 from surface at 90 contours A8 | A10 | A12 | A15 bodies 2 3 1 4 5
sketch "Skizze29" plane through (185, 0, 0) normal (1, 0, 0) x (0, 0, -1)
  line L0 (29.4, 0) -> (160.2, 0)
  line L1 (160.2, 0) -> (160.2, 90)
  line L2 (160.2, 90) -> (29.4, 90)
  line L3 (29.4, 90) -> (29.4, 0)
  circle A0 centre (59.4, 38.5) radius 10
  circle A1 centre (130.2, 38.5) radius 10
  dimension "d671" = 20
  dimension "d672" = 20
  dimension "d673" = 38.5
  dimension "d674" = 30
  dimension "d675" = 30
  constraint horizontal A0.centre A1.centre
  measures "d671" diameter of A0
  measures "d672" diameter of A1
  measures "d673" distance of L0 A0.centre
  measures "d674" distance of L3 A0.centre
  measures "d675" distance of L1 A1.centre
extrude "Extrusion62" cut sketch "Skizze29" against normal up to surface (2.4 mm away) contours A0 | A1 bodies 5
extrude "Extrusion22" add sketch "Skizze9" along normal blind 50 from surface at 10 separate body contours L4 L5 L6 L7 L10 L11 L14 L21 L22 L25 | L6 L8 L10 L11 L29 | L6 L20 L21 L22 L24 | L6 L8 L9 L10 L15 L29 L30 | L6 L13 L20 L22 L23 L24 L25 L27 | L6 L9 L12 L14 L15 L28 L30 | L6 L12 L13 L14 L23 L25 L26 L27 | L6 L12 L14 L26 L28 | A0 | A1 | A2 | A3 | A4 | A5 | A6 | A7 makes body 7
sketch "Skizze12" plane through (0, 0, -156.8) normal (0, 0, -1) x (-1, 0, 0)
  line L0 (-160, 10) -> (-13, 10)
  line L1 (-13, 10) -> (-13, 60)
  line L2 (-13, 60) -> (-160, 60)
  line L3 (-160, 60) -> (-160, 10)
  line L4 (-84.55, 10) -> (-68.35, 10)
  line L5 (-68.35, 10) -> (-68.35, 25)
  line L6 (-68.35, 25) -> (-84.55, 25)
  line L7 (-84.55, 25) -> (-84.55, 10)
  line L8 (-68.35, 10) -> (-49.9, 10)
  line L9 (-49.9, 10) -> (-49.9, 22)
  line L10 (-49.9, 22) -> (-68.35, 22)
  line L11 (-68.35, 22) -> (-68.35, 10)
  line L12 (-49.9, 10) -> (-31.68, 10)
  line L13 (-31.68, 10) -> (-31.68, 20)
  line L14 (-31.68, 20) -> (-49.9, 20)
  line L15 (-49.9, 20) -> (-49.9, 10)
  line L16 (-48.9, 20) -> (-48.9, 10)
  line L17 (-50.9, 22) -> (-50.9, 10)
  line L18 (-67.35, 22) -> (-67.35, 10)
  line L19 (-69.35, 25) -> (-69.35, 10)
  point P0 (-84.55, 0)
  point P1 (-68.35, 0)
  point P2 (-49.9, 0)
  point P3 (-31.68, 0)
  point P4 (-48.9, 0)
  point P5 (-50.9, 0)
  point P6 (-67.35, 0)
  point P7 (-69.35, 0)
  dimension "d230" = 15
  dimension "d231" = 12
  dimension "d234" = 10
  constraint horizontal L4
  constraint vertical L5
  constraint horizontal L6
  constraint vertical L7
  constraint coincident L0 L4.start
  constraint horizontal L8
  constraint vertical L9
  constraint horizontal L10
  constraint vertical L11
  constraint coincident L0 L4.end
  constraint horizontal L12
  constraint vertical L13
  constraint horizontal L14
  constraint vertical L15
  constraint coincident L0 L8.end
  constraint coincident L7 P0
  constraint coincident L5 P1
  constraint coincident L11 P1
  constraint coincident L9 P2
  constraint coincident L15 P2
  constraint coincident L13 P3
  constraint coincident L14 L16.start
  constraint coincident L12 L16.end
  constraint perpendicular L12 L16
  constraint coincident L16 P4
  constraint vertical L17
  constraint coincident L10 L17.start
  constraint coincident L17 P5
  constraint vertical L18
  constraint coincident L10 L18.start
  constraint coincident L18 P6
  constraint vertical L19
  constraint coincident L6 L19.start
  constraint coincident L19 P7
  constraint coincident L4 L19.end
  constraint coincident L8 L18.end
  constraint coincident L8 L17.end
  measures "d230" distance of L4.start L6.end
  measures "d231" distance of L4.end L10.end
  measures "d234" distance of L12 L14
extrude "Extrusion24" cut sketch "Skizze12" along normal up to surface (2.4 mm away) from surface at 1 contours L0 L4 L6 L7 L19 | L0 L8 L10 L17 L18 | L0 L12 L13 L14 L16 bodies 5
move_body "Verschieben2" bodies 1 3 2 to x (1, 0, 0) y (0, 1, 0) z (0, 0, 1) at (0, 26, 0)
sketch "Skizze16" plane through (0, 0, -29.4) normal (0, 0, 1) x (1, 0, 0)
  line L0 (-8.8, 0) -> (122.3, 0)
  line L1 (122.3, 0) -> (122.3, 91.8)
  line L2 (122.3, 91.8) -> (-8.8, 91.8)
  line L3 (-8.8, 91.8) -> (-8.8, 0)
  circle A0 centre (57.3, 47.5) radius 10
  line L4 (122.3, 0) -> (122.3, 91.8)
  line L5 (-8.8, 91.8) -> (-8.8, 0)
  line L6 (122.3, 0) -> (-8.8, 0)
  line L7 (160.2, 0) -> (29.4, 0)
  line L8 (160.2, -2.4) -> (160.2, 0)
  line L9 (29.4, 0) -> (29.4, -2.4)
  line L10 (29.4, -2.4) -> (160.2, -2.4)
  line L11 (-9.4, 0) -> (185, 0)
  line L12 (185, 0) -> (185, 90)
  line L13 (185, 90) -> (-9.4, 90)
  line L14 (-9.4, 90) -> (-9.4, 0)
  dimension "d277" = 20
  dimension "d278" = 65
  dimension "d280" = 47.5
  measures "d277" diameter of A0
  measures "d278" distance of A0.centre L4
  measures "d280" distance of A0.centre L6
extrude "Extrusion26" cut sketch "Skizze16" along normal up to surface (24.8 mm away) from surface at -2.4 contours A0 bodies 1 5